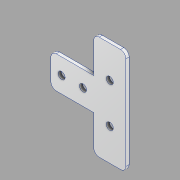
# Autodesk Inventor part: bogie_mount
Saved by Autodesk Inventor 2021.3 (Build 253353000, 353)
## iProperties
Created: 2021-07-08
Part Number: bogie_mount
Material: アルミニウム 6061
Document SubType Name: Modeling
Designer: gisen
Density: 2.7 g/cm^3
Appearance: アルミニウム - フラット
Author: gisen
Autodesk Inventor part; units mm, degrees
ref_plane "YZ Plane" through (0, 0, 0) normal (1, 0, 0) x (0, 1, 0)
ref_plane "XZ Plane" through (0, 0, 0) normal (0, 1, 0) x (-1, 0, 0)
ref_plane "XY Plane" through (0, 0, 0) normal (0, 0, 1) x (1, 0, 0)
ref_plane "作業平面1" through (0, 0, 0) normal (0, 0, 1) x (1, 0, 0)
sketch "スケッチ2" plane through (0, 0, 0) normal (0, 0, 1) x (1, 0, 0)
  line L0 (0, 0) -> (7.35, 0) construction
  line L1 (7.35, 0) -> (7.35, 50) construction
  line L2 (0, 50) -> (7.35, 50) construction
  line L3 (0, 0) -> (0, 50) construction
  line L4 (-0.5, 0) -> (-0.5, 50) construction
  line L5 (19.5, 0) -> (19.5, 50) construction
  line L6 (139.5, 0) -> (139.5, -3) construction
  line L7 (139.5, 0) -> (4.5, 0) construction
  line L8 (4.5, -3) -> (4.5, 0) construction
  line L9 (139.5, -3) -> (4.5, -3) construction
  line L10 (139.5, 53) -> (139.5, 50) construction
  line L11 (4.5, 53) -> (139.5, 53) construction
  line L12 (4.5, 50) -> (4.5, 53) construction
  line L13 (4.5, 50) -> (139.5, 50) construction
  line L14 (-0.632, 5) -> (-130.632, 5) construction
  line L15 (-0.632, 45) -> (-130.632, 45) construction
  line L16 (-40.5, 33.5) -> (-40.5, 63.5)
  line L17 (-40.5, 63.5) -> (-0.5, 63.5)
  line L18 (-0.5, 63.5) -> (-0.5, 5)
  circle A0 centre (14.5, 30) radius 3.3
  circle A1 centre (14.5, 67) radius 3.3
  circle A2 centre (-30.5, 48.5) radius 3.3
  circle A3 centre (-10.5, 48.5) radius 3.3
  line L19 (-40.5, 33.5) -> (-0.5, 33.5)
  line L20 (-0.5, 0) -> (29.5, 0)
  line L21 (29.5, 0) -> (29.5, 97)
  line L22 (29.5, 97) -> (-0.5, 97)
  line L23 (-0.5, 97) -> (-0.5, 0)
  point P0 (9.5, 35)
  point P1 (-0.5, 33.5)
  point P2 (-0.5, 63.5)
  point P3 (-0.5, 5)
  dimension "d1" = 40
  dimension "d2" = 30
  dimension "d4" = 50
  dimension "d5" = 30
  dimension "d13" = 6.6
  dimension "d17" = 6.6
  dimension "d19" = 10
  dimension "d20" = 6.6
  dimension "d22" = 10
  dimension "d23" = 6.6
  dimension "d27" = 33.5
  dimension "d29" = 15
  dimension "d30" = 15
  dimension "d31" = 30
  dimension "d32" = 97
  dimension "d33" = 15
  dimension "d34" = 15
  dimension "d35" = 30
  constraints: 16 end point, 4 centre point, 4 parallel, 2 perpendicular, 1 coincident, 1 collinear, 1 horizontal, 1 point on line
  measures "d1" distance of L16.end L17.end
  measures "d2" distance of L16.start L16.end
  measures "d4" distance between parallel lines of L2 L0
  measures "d5" distance from line of L7 point (14.5, 30)
  measures "d13" diameter of A0
  measures "d17" diameter of A2
  measures "d19" distance from line of L16 A2.centre
  measures "d20" diameter of A3
  measures "d22" distance from line of L4 A3.centre
  measures "d23" diameter of A1
  measures "d27" distance between parallel lines of L7 L19
  measures "d29" distance from line of L19 A3.centre
  measures "d30" distance from line of L19 A2.centre
  measures "d31" distance of L22.end L21.end
  measures "d32" distance of L21.end L20.end
  measures "d33" distance from line of L21 A0.centre
  measures "d34" distance from line of L21 A1.centre
  measures "d35" distance from line of L22 A1.centre
extrude "押し出し1" add sketch "スケッチ2" along normal blind 3
fillet "フィレット1" radius 5 6 edges at (-40.5, 33.5, 1.5) (-40.5, 63.5, 1.5) (-0.5, 0, 1.5) (29.5, 0, 1.5) (-0.5, 97, 1.5) (29.5, 97, 1.5)
equation "\"d22\" = d19"
equation "\"d23\" = d13"
equation "\"d27\" = -0.5 * d2 + 0.5 * d32"
equation "\"d29\" = 0.5 * d2"
equation "\"d30\" = d29"
equation "\"d33\" = 0.5 * d31"
equation "\"d34\" = d33"
